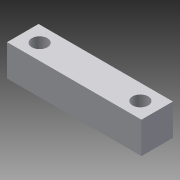
# Autodesk Inventor part: yCarBeltTensioner
Saved by Autodesk Inventor 2013 (Build 170138000, 138)
## iProperties
Created: 2015-01-14
Part Number: yCarBeltTensioner
Material: Generic
Document SubType Name: Modeling
Designer: dzban
Density: 1 g/cm^3
Author: dzban
Autodesk Inventor part; units mm, degrees
ref_plane "YZ Plane" through (0, 0, 0) normal (1, 0, 0) x (0, 1, 0)
ref_plane "XZ Plane" through (0, 0, 0) normal (0, 1, 0) x (-1, 0, 0)
ref_plane "XY Plane" through (0, 0, 0) normal (0, 0, 1) x (1, 0, 0)
sketch "Sketch1" plane through (0, 0, 0) normal (0, 0, 1) x (1, 0, 0)
  circle A0 centre (-16.1429, 1.3714) radius 1.5
  circle A1 centre (3.0571, 1.3714) radius 1.5
  line L0 (6.2571, 4.3714) -> (-19.3429, 4.3714)
  line L1 (-19.3429, 4.3714) -> (-19.3429, -1.6286)
  line L2 (-19.3429, -1.6286) -> (6.2571, -1.6286)
  line L3 (6.2571, -1.6286) -> (6.2571, 4.3714)
  point P0 (0, 0)
  point P1 (0, 0)
  constraints: 8 end point, 2 centre point
extrude "Extrusion1" add sketch "Sketch1" along normal blind 6
body "Solid1"
